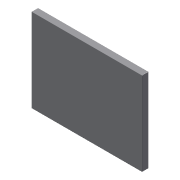
# Autodesk Inventor part: BeddingStopper
Saved by Autodesk Inventor 2016 (Build 200138000, 138)
## iProperties
Created: 2018-04-09
Part Number: BeddingStopper
Material: Generic
Document SubType Name: Sheet Metal
Designer: reinert
Density: 1 g/cm^3
Sheet Metal Rule: Default_mm
Appearance: Default
Author: reinert
Autodesk Inventor part; units mm, degrees
note: some values were not read from the file. Chosen so that the rebuilt part matches the saved one: corner form of "Plate2".
ref_plane "YZ Plane" through (0, 0, 0) normal (1, 0, 0) x (0, 1, 0)
ref_plane "XZ Plane" through (0, 0, 0) normal (0, 1, 0) x (-1, 0, 0)
ref_plane "XY Plane" through (0, 0, 0) normal (0, 0, 1) x (1, 0, 0)
sketch "Sketch1" plane through (0, 0, 0) normal (0, 1, 0) x (-1, 0, 0)
  line L0 (0, 0) -> (700, 0)
  line L1 (700, 0) -> (700, -529.8)
  line L2 (700, -529.8) -> (0, -529.8)
  line L3 (0, -529.8) -> (0, 0)
  dimension "d0" = 700
  dimension "d1" = 529.8
  measures "d0" distance of L1.end L2.end
  measures "d1" distance of L0.end L1.end
extrude "Plate1" add sketch "Sketch1" along normal blind 0.5
sketch "Sketch2" plane through (-700, 0, -529.3) normal (0, 0, -1) x (-1, 0, 0)
  line L0 (-700, 0) -> (0, 0)
  line L1 (0, 0) -> (0, 40)
  line L2 (0, 40) -> (-700, 40)
  line L3 (-700, 40) -> (-700, 0)
  constraints: 6 end point, 1 horizontal, 1 perpendicular, 1 vertical
edge flange "Flange1" height 40 angle 90 thickness 0.5 bend radius 0.5 thickness toward (0, 0, -1) relief tear relief width 0.5 relief depth 0.25 corner gap 0.5 corner form 2 edges at (-350, 0.5, -529.8) (0, 0.5, -264.9) (-350, 0.5, 0) (-700, 0.5, -264.9) wall of the first edge with corners at (0, 0, -529.3) (-700, 0, -529.3) (-700, 40, -529.3) (0, 40, -529.3)
bend "Bend1"
corner "Corner1"
equation "\"d3\" = BendReliefWidth"
equation "\"d4\" = BendReliefDepth"
equation "\"d5\" = MinimumRemnant"
equation "\"d6\" = BendRadius"
equation "\"d9\" = BendRadius"
equation "\"d10\" = CornerReliefSize"
equation "\"d11\" = GapSize"
equation "\"d12\" = JacobiRadiusSize"
equation "\"BendRadius\" = Thickness"
equation "\"BendReliefWidth\" = Thickness"
equation "\"BendReliefDepth\" = 0.5 * Thickness"
equation "\"CornerReliefSize\" = 4 * Thickness"
equation "\"MinimumRemnant\" = 2 * Thickness"
equation "\"TransitionRadius\" = BendRadius"
equation "\"JacobiRadiusSize\" = BendRadius"
equation "\"GapSize\" = Thickness"
equation "\"d2\" = BendRadius"
equation "\"Thickness\" = 0.5"
body "Solid1"
